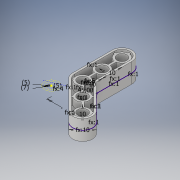
# Autodesk Inventor part: Bent beam 5-135
Saved by Autodesk Inventor 2019 (Build 230136000, 136)
## iProperties
Created: 2019-01-29
Part Number: Bent beam 5-135
Material: Generic
Document SubType Name: Modeling
Designer: Varga Daniel
Density: 1 g/cm^3
Appearance: Default
Author: Varga Daniel
Autodesk Inventor part; units mm, degrees
ref_plane "YZ Plane" through (0, 0, 0) normal (1, 0, 0) x (0, 1, 0)
ref_plane "XZ Plane" through (0, 0, 0) normal (0, 1, 0) x (-1, 0, 0)
ref_plane "XY Plane" through (0, 0, 0) normal (0, 0, 1) x (1, 0, 0)
derived "Base_part.ipt"
sketch "Sketch1" plane through (0, 0, 0) normal (0, 1, 0) x (-1, 0, 0)
  line L0 (5, 0) -> (25, 0)
  line L1 (30, 5) -> (30, 25)
  line L2 (25, 30) -> (5, 30)
  line L3 (0, 25) -> (0, 5)
  line L4 (5, 29) -> (25, 29)
  line L5 (29, 25) -> (29, 5)
  line L6 (25, 1) -> (5, 1)
  line L7 (1, 5) -> (1, 25)
  circle A0 centre (5, 5) radius 2.5
  circle A1 centre (5, 5) radius 3.5
  arc A2 (25, 0) -> (30, 5) centre (25, 5) ccw
  arc A3 (30, 25) -> (25, 30) centre (25, 25) ccw
  arc A4 (5, 30) -> (0, 25) centre (5, 25) ccw
  arc A5 (0, 5) -> (5, 0) centre (5, 5) ccw
  arc A6 (1, 5) -> (5, 1) centre (5, 5) ccw
  arc A7 (5, 29) -> (1, 25) centre (5, 25) ccw
  arc A8 (29, 25) -> (25, 29) centre (25, 25) ccw
  arc A9 (25, 1) -> (29, 5) centre (25, 5) ccw
  line L8 (49.1041, 15) -> (-27.081, 15) construction
  line L9 (31.1478, 10) -> (-2.4877, 10) construction
  line L10 (-2.8604, 5) -> (35.495, 5) construction
  line L11 (5, -2.5736) -> (5, 36.7522) construction
  line L12 (15, -1.4978) -> (15, 34.8784) construction
  line L13 (1.5359, 5.5) -> (1, 5.5)
  line L14 (1.5359, 4.5) -> (1.0314, 4.5)
  line L15 (28.9686, 4.5) -> (8.4641, 4.5)
  line L16 (29, 5.5) -> (8.4641, 5.5)
  line L17 (4.5, 1.5359) -> (4.5, 1.0314)
  line L18 (5.5, 1.5359) -> (5.5, 1)
  line L19 (29, 10.5) -> (1, 10.5)
  line L20 (29, 9.5) -> (1, 9.5)
  line L21 (4.5, 28.9686) -> (4.5, 10.5)
  line L22 (4.5, 9.5) -> (4.5, 8.4641)
  line L23 (5.5, 29) -> (5.5, 10.5)
  line L24 (5.5, 9.5) -> (5.5, 8.4641)
  point P0 (0, 0)
  point P1 (30, 30)
  point P2 (0, 30)
  point P3 (5, 25)
sketch "Sketch2" plane through (0, 0, 0) normal (0, 1, 0) x (-1, 0, 0)
  line L0 (-9.8186, -3.1319) -> (-9.8186, -21.0609)
  line L1 (0.1814, -1.0609) -> (0.1814, -21.0609)
  line L2 (0.1814, -21.0609) -> (-9.8186, -21.0609) construction
  line L3 (-0.8186, -1.0609) -> (-0.8186, -21.0609)
  line L4 (-8.8186, -3.1319) -> (-8.8186, -21.0609)
  line L5 (-4.8186, -1.0609) -> (-4.8186, -21.0609) construction
  line L6 (-9.8186, -3.1319) -> (-22.4963, 9.5457)
  line L7 (-21.7892, 10.2528) -> (-9.1115, -2.4248)
  line L8 (-4.8186, -1.0609) -> (-2.3335, -3.5461) construction
  line L9 (-9.8186, -3.1319) -> (9.7269, 4.9641) construction
  arc A0 (-8.8186, -3.1319) -> (-9.1115, -2.4248) centre (-9.8186, -3.1319) ccw
  arc A1 (0.1814, -1.0609) -> (-1.2831, 2.4747) centre (-4.8186, -1.0609) ccw
  line L10 (-1.2831, 2.4747) -> (-15.4252, 16.6168)
  line L11 (-1.9902, 1.7675) -> (-16.1324, 15.9097)
  arc A2 (-0.8186, -1.0609) -> (-1.9902, 1.7675) centre (-4.8186, -1.0609) ccw
  line L12 (-15.4252, 16.6168) -> (-22.4963, 9.5457) construction
  circle A3 centre (-4.8186, -1.0609) radius 2.5
  circle A4 centre (-4.8186, -1.0609) radius 3.5
  arc A5 (-9.8186, -21.0609) -> (0.1814, -21.0609) centre (-4.8186, -21.0609) ccw
  arc A6 (-8.8186, -21.0609) -> (-0.8186, -21.0609) centre (-4.8186, -21.0609) ccw
  circle A7 centre (-11.8897, 6.0102) radius 2.5
  circle A8 centre (-11.8897, 6.0102) radius 3.5
  arc A9 (-15.4252, 16.6168) -> (-22.4963, 9.5457) centre (-18.9608, 13.0813) ccw
  arc A10 (-16.1324, 15.9097) -> (-21.7892, 10.2528) centre (-18.9608, 13.0813) ccw
  circle A11 centre (-18.9608, 13.0813) radius 2.5
  circle A12 centre (-18.9608, 13.0813) radius 3.5
  circle A13 centre (-4.8186, -11.0609) radius 2.5
  circle A14 centre (-4.8186, -11.0609) radius 3.5
  circle A15 centre (-4.8186, -21.0609) radius 2.5
  circle A16 centre (-4.8186, -21.0609) radius 3.5
  line L13 (-4.3186, -4.525) -> (-4.3186, -7.5968)
  line L14 (-5.3186, -7.5968) -> (-5.3186, -4.525)
  line L15 (-5.3186, -14.525) -> (-5.3186, -17.5968)
  line L16 (-4.3186, -14.525) -> (-4.3186, -17.5968)
  line L17 (-5.3186, -25.0295) -> (-5.3186, -24.525)
  line L18 (-4.3186, -25.0295) -> (-4.3186, -24.525)
  line L19 (-7.6217, 1.0351) -> (-9.7938, 3.2071)
  line L20 (-9.0867, 3.9143) -> (-6.9146, 1.7422)
  line L21 (-14.6928, 8.1061) -> (-16.8648, 10.2782)
  line L22 (-16.1577, 10.9853) -> (-13.9857, 8.8132)
  line L23 (-21.7638, 15.1772) -> (-22.1206, 15.5339)
  line L24 (-21.0567, 15.8843) -> (-21.4135, 16.2411)
  line L25 (-4.8186, -11.0609) -> (-8.8186, -11.0609) construction
  line L26 (-8.2827, -11.5609) -> (-8.8186, -11.5609)
  line L27 (-8.2827, -10.5609) -> (-8.8186, -10.5609)
  line L28 (-1.3545, -11.5609) -> (-0.8186, -11.5609)
  line L29 (-1.3545, -10.5609) -> (-0.8186, -10.5609)
  line L30 (-8.2827, -21.5609) -> (-8.7873, -21.5609)
  line L31 (-8.2827, -20.5609) -> (-8.8186, -20.5609)
  line L32 (-1.3545, -21.5609) -> (-0.85, -21.5609)
  line L33 (-0.8186, -20.5609) -> (-1.3545, -20.5609)
  line L34 (-11.8897, 6.0102) -> (-14.7181, 3.1818) construction
  line L35 (-14.3646, 2.8282) -> (-13.9857, 3.2071)
  line L36 (-14.6928, 3.9143) -> (-15.0717, 3.5353)
  line L37 (-9.0867, 8.1061) -> (-8.7077, 8.4851)
  line L38 (-9.7938, 8.8132) -> (-9.4148, 9.1922)
  line L39 (-21.4357, 9.8993) -> (-21.0567, 10.2782)
  line L40 (-21.7638, 10.9853) -> (-22.1206, 10.6286)
  line L41 (-16.1577, 15.1772) -> (-15.7788, 15.5561)
  line L42 (-16.8648, 15.8843) -> (-16.5081, 16.2411)
  line L43 (-0.9608, -0.0041) -> (-1.4269, -0.1972)
  line L44 (-1.3435, 0.9198) -> (-1.8096, 0.7267)
  circle A17 centre (5, 5) radius 2.5 construction
  circle A18 centre (5, 5) radius 3.5 construction
  point P0 (-5.3186, 2.4032)
  point P1 (-4.3186, 2.4032)
  point P2 (-2.7227, -3.8639)
  point P3 (-2.0156, -3.1568)
  dimension "d19" = 7
  dimension "d5" = 10
  dimension "d7" = 1
  dimension "d8" = 1
  dimension "d9" = 135
  dimension "d10" = 1
  dimension "d11" = 1
  dimension "d12" = 5
  dimension "d13" = 10
  dimension "d14" = 1
  dimension "d16" = 5
  dimension "d17" = 4
  dimension "d18" = 5
  dimension "d50" = 10
  dimension "d64" = 10
  dimension "d71" = 10
  dimension "d78" = 10
  dimension "d83" = 1
  dimension "d84" = 1
  dimension "d85" = 1
  dimension "d86" = 1
  dimension "d87" = 1
  dimension "d88" = 1
  dimension "d96" = 1
  dimension "d105" = 5
  dimension "d106" = 7
  constraints: 90 end point, 24 point on circle, 22 parallel, 19 point on line, 16 collinear, 12 centre point, 8 coincident, 8 tangent, 7 vertical, 4 perpendicular, 3 midpoint, 76 other
  measures "d5" distance between parallel lines of L0 L1
  measures "d7" distance between parallel lines of L1 L3
  measures "d8" distance between parallel lines of L0 L4
  measures "d9" angle of L5 L8
  measures "d10" distance between parallel lines of L6 L7
  measures "d11" radius of A0
  measures "d12" distance between parallel lines of L8 L6
  measures "d13" distance between parallel lines of L10 L6
  measures "d14" distance between parallel lines of L11 L10
  measures "d16" radius of A1
  measures "d17" radius of A2
  measures "d18" diameter of A3
  measures "d50" distance of A3.centre A7.centre
  measures "d64" distance of A7.centre A11.centre
  measures "d71" distance of A3.centre A13.centre
  measures "d78" distance of A13.centre A15.centre
  measures "d83" distance between parallel lines of L14 L13
  measures "d84" distance between parallel lines of L20 L19
  measures "d85" distance between parallel lines of L27 L26
  measures "d86" distance between parallel lines of L31 L30
  measures "d87" distance between parallel lines of L35 L36
  measures "d88" distance between parallel lines of L40 L39
  measures "d96" distance between parallel lines of L44 L43
  measures "d105" diameter of A17
  measures "d106" diameter of A18
extrude "Extrusion1" add sketch "Sketch2" along normal blind 5 contours L6 A9 L10 A1 L1 A5 L0
extrude "Extrusion2" add sketch "Sketch2" against normal blind 5 contours L6 A9 L10 A1 L1 A5 L0
extrude "Extrusion4" add sketch "Sketch2" along normal blind 4.2 contours L3 L28 A14 L29 | L43 A4 L44 A2 | A14 | A4 | L3 A6 L32 A16 L33 | A14 L14 A4 L13 | A16 | L16 A16 L15 A14 | L37 A8 L38 L11 | A4 L19 A8 L20 | A14 L26 L4 L27 | A8 | A6 L17 A16 L18 | L41 A12 L42 A10 L11 | A16 L30 A6 L4 L31 | A12 | A8 L21 A12 L22 | L35 L7 L36 A8 | L24 A12 L23 A10 | L39 L7 A10 L40 A12
extrude "Extrusion5" add sketch "Sketch2" against normal blind 4.2 contours L3 L28 A14 L29 | L43 A4 L44 A2 | A14 | A4 | L3 A6 L32 A16 L33 | A14 L14 A4 L13 | A16 | L16 A16 L15 A14 | L37 A8 L38 L11 | A4 L19 A8 L20 | A14 L26 L4 L27 | A8 | A6 L17 A16 L18 | L41 A12 L42 A10 L11 | A16 L30 A6 L4 L31 | A12 | A8 L21 A12 L22 | L35 L7 L36 A8 | L24 A12 L23 A10 | L39 L7 A10 L40 A12
extrude "Extrusion6" add sketch "Sketch2" along normal blind 0.5 contours L3 L29 A14 L13 A4 L43 A2 | L3 L33 A16 L16 A14 L28 | L44 A4 L20 A8 L37 L11 A2 | A14 L27 L4 A0 L7 L35 A8 L19 A4 L14 | A6 L18 A16 L32 | L15 A16 L31 L4 L26 A14 | L38 A8 L22 A12 L41 L11 | A6 L30 A16 L17 | L42 A12 L24 A10 | A8 L36 L7 L39 A12 L21 | L23 A12 L40 A10
extrude "Extrusion7" add sketch "Sketch2" against normal blind 0.5 contours L3 L29 A14 L13 A4 L43 A2 | L3 L33 A16 L16 A14 L28 | L44 A4 L20 A8 L37 L11 A2 | A14 L27 L4 A0 L7 L35 A8 L19 A4 L14 | A6 L18 A16 L32 | L15 A16 L31 L4 L26 A14 | L38 A8 L22 A12 L41 L11 | A6 L30 A16 L17 | L42 A12 L24 A10 | A8 L36 L7 L39 A12 L21 | L23 A12 L40 A10
equation "\"d7\" = Wall_thickness"
equation "\"d8\" = d7"
equation "\"d10\" = d7"
equation "\"d11\" = d7"
equation "\"d12\" = 0.5 * d5"
equation "\"d13\" = d5"
equation "\"d14\" = d7"
equation "\"d17\" = d16 - d7"
equation "\"d83\" = Inner_route_thickness"
equation "\"d84\" = Inner_route_thickness"
equation "\"d85\" = Inner_route_thickness"
equation "\"d86\" = Inner_route_thickness"
equation "\"d87\" = Inner_route_thickness"
equation "\"d88\" = Inner_route_thickness"
equation "\"d89\" = 0.5 * Overall_height"
equation "\"d91\" = 0.5 * Overall_height"
equation "\"Wall_thickness\" = 1"
equation "\"Inner_route_thickness\" = 1"
equation "\"Overall_height\" = 10"
body "Solid1"
